Autodesk Inventor part; units mm, degrees
(part 2 of 2)
  line L793 (-106453, -86326.2124) -> (-106453, -83926.2124)
  line L794 (-106453, -83926.2124) -> (-106353, -83926.2124)
  line L795 (-106353, -83926.2124) -> (-106353, -90167.9126)
  line L796 (-106353, -90167.9126) -> (-97738.8492, -90167.9126)
  line L797 (-106453, -82706.2124) -> (-106353, -82706.2124)
  line L798 (-106353, -82706.2124) -> (-106353, -82456.2124)
  line L799 (-106453, -82706.2124) -> (-106453, -82206.2124)
  line L800 (-106353, -82456.2124) -> (-104713, -82456.2124)
  line L801 (-104713, -82456.2124) -> (-104713, -83516.2124)
  line L802 (-104713, -83516.2124) -> (-103563, -83516.2124)
  line L803 (-103563, -83516.2124) -> (-103563, -82456.2124)
  line L804 (-103563, -82456.2124) -> (-98350.4288, -82456.2124)
  line L805 (-97738.8492, -90167.9126) -> (-98350.4288, -82456.2124)
  line L806 (-106453, -82206.2124) -> (-104713, -82206.2124)
  line L807 (-104713, -82206.2124) -> (-104713, -82106.2124)
  line L808 (-104713, -82106.2124) -> (-103563, -82106.2124)
  line L809 (-103563, -82106.2124) -> (-103563, -82206.2124)
  line L810 (-103563, -82206.2124) -> (-101863, -82206.2124)
  line L811 (-107613, -65817.8595) -> (-107513, -65817.8595)
  line L812 (-107513, -65817.8595) -> (-107513, -65467.8595)
  line L813 (-107513, -65467.8595) -> (-104713, -65467.8595)
  line L814 (-104713, -65467.8595) -> (-104713, -66447.8595)
  line L815 (-104713, -66447.8595) -> (-103563, -66447.8595)
  line L816 (-103563, -66447.8595) -> (-103563, -65467.8595)
  line L817 (-107613, -67037.8595) -> (-107613, -67637.8595)
  line L818 (-107613, -67637.8595) -> (-108513, -70077.1217)
  line L819 (-107613, -67037.8595) -> (-107513, -67037.8595)
  line L820 (-107513, -67037.8595) -> (-107513, -70077.1217)
  line L821 (-108513, -70077.1217) -> (-108513, -71877.1217)
  line L822 (-101863, -82206.2124) -> (-101863, -81606.2124)
  line L823 (-101863, -81606.2124) -> (-101763, -81606.2124)
  line L824 (-101763, -81606.2124) -> (-101763, -82206.2124)
  line L825 (-101763, -82206.2124) -> (-98119.4702, -82206.2124)
  line L826 (-98365.317, -79106.2124) -> (-101763, -79106.2124)
  line L827 (-101763, -79106.2124) -> (-101763, -79706.2124)
  line L828 (-101763, -79706.2124) -> (-101863, -79706.2124)
  line L829 (-101963, -79106.2124) -> (-101963, -79056.2124)
  line L830 (-101963, -79056.2124) -> (-103013, -79056.2124)
  line L831 (-103013, -79056.2124) -> (-103013, -78956.2124)
  line L832 (-98635.9282, -78856.2124) -> (-99052.2817, -73606.2124)
  line L833 (-103963, -79056.2124) -> (-103963, -74806.2124)
  line L834 (-103963, -79056.2124) -> (-107463, -79056.2124)
  line L835 (-107463, -78956.2124) -> (-107463, -79056.2124)
  line L836 (-108413, -79056.2124) -> (-108513, -79056.2124)
  line L837 (-108513, -79056.2124) -> (-108513, -74016.2124)
  line L838 (-108413, -73606.2124) -> (-108413, -79056.2124)
  line L839 (-108513, -71877.1217) -> (-108413, -71877.1217)
  line L840 (-101863, -79106.2124) -> (-101963, -79106.2124)
  line L841 (-101863, -79706.2124) -> (-101863, -79106.2124)
  line L842 (-103013, -78956.2124) -> (-101963, -78956.2124)
  line L843 (-101963, -78956.2124) -> (-101963, -78856.2124)
  line L844 (-101963, -78856.2124) -> (-98635.9282, -78856.2124)
  line L845 (-107463, -78956.2124) -> (-104063, -78956.2124)
  line L846 (-108413, -73356.2124) -> (-108413, -73097.1217)
  line L847 (-108413, -73097.1217) -> (-108513, -73097.1217)
  line L848 (-108513, -73097.1217) -> (-108513, -74016.2124)
  line L849 (-108413, -73606.2124) -> (-104713, -73606.2124)
  line L850 (-104713, -73606.2124) -> (-104713, -74806.2124)
  line L851 (-104713, -74806.2124) -> (-103413, -74806.2124)
  line L852 (-104063, -74806.2124) -> (-104063, -78956.2124)
  line L853 (-103413, -74806.2124) -> (-103413, -73606.2124)
  line L854 (-103413, -73606.2124) -> (-99052.2817, -73606.2124)
  line L855 (-99072.108, -73356.2124) -> (-99697.6971, -65467.8595)
  line L856 (-104713, -70227.1217) -> (-104713, -73356.2124)
  line L857 (-107513, -70077.1217) -> (-104563, -70077.1217)
  line L858 (-108413, -71877.1217) -> (-108413, -70227.1217)
  line L859 (-108413, -70227.1217) -> (-104713, -70227.1217)
  line L860 (-108513, -70077.1217) -> (-107513, -70077.1217) construction
  line L861 (-104563, -70077.1217) -> (-104563, -73356.2124)
  line L862 (-99072.108, -73356.2124) -> (-104563, -73356.2124)
  line L863 (-104713, -73356.2124) -> (-108413, -73356.2124)
  line L864 (-99697.6971, -65467.8595) -> (-103563, -65467.8595)
  line L865 (-104613, -99029.6129) -> (-104613, -98659.6129)
  line L866 (-104613, -98659.6129) -> (-103653, -98659.6129)
  line L867 (-106353, -99029.6129) -> (-104613, -99029.6129)
  line L868 (-103653, -99029.6129) -> (-97036.0684, -99029.6129)
  line L869 (-103653, -98659.6129) -> (-103653, -99029.6129)
  line L870 (-92256.354, -106329.6129) -> (-92256.354, -78829.6129)
  line L871 (-96222.2151, -106129.6129) -> (-92456.354, -106129.6129)
  line L872 (-96206.354, -106329.6129) -> (-92256.354, -106329.6129)
  line L873 (-92456.354, -106129.6129) -> (-92456.354, -78877.5442)
  line L874 (-99463, -65217.8595) -> (-99178.2074, -65217.8595)
  line L875 (-99450.8774, -65417.8595) -> (-99300.8774, -65417.8595)
  line L876 (-92456.354, -78877.5442) -> (-99300.8774, -65417.8595)
  line L877 (-92256.354, -78829.6129) -> (-99178.2074, -65217.8595)
  line L878 (-92456.354, -99487.1129) -> (-93271.354, -99487.1129)
  line L879 (-93271.354, -99487.1129) -> (-93271.354, -98672.1129)
  line L880 (-93271.354, -98672.1129) -> (-92456.354, -98672.1129)
  line L881 (-92456.354, -98672.1129) -> (-92456.354, -99487.1129)
  line L882 (-92456.354, -99487.1129) -> (-93271.354, -98672.1129) construction
  line L883 (-93271.354, -99487.1129) -> (-92456.354, -98672.1129) construction
  line L884 (-92456.354, -90987.1129) -> (-93271.354, -90987.1129)
  line L885 (-93271.354, -90987.1129) -> (-93271.354, -90172.1129)
  line L886 (-93271.354, -90172.1129) -> (-92456.354, -90172.1129)
  line L887 (-92456.354, -90172.1129) -> (-92456.354, -90987.1129)
  line L888 (-92456.354, -82487.1129) -> (-93271.354, -82487.1129)
  line L889 (-93271.354, -82487.1129) -> (-93271.354, -81672.1129)
  line L890 (-93271.354, -81672.1129) -> (-92456.354, -81672.1129)
  line L891 (-92456.354, -81672.1129) -> (-92456.354, -82487.1129)
  line L892 (-48823, -52627.8595) -> (-48823, -52097.8595)
  line L893 (-48823, -52097.8595) -> (-42123, -52097.8595)
  line L894 (-42123, -52097.8595) -> (-42123, -52627.8595)
  line L895 (-38789.6466, -50375.6793) -> (-39177.876, -49986.0924)
  line L896 (-39177.876, -49986.0924) -> (-40629.9726, -51433.1291)
  line L897 (-40629.9726, -51433.1291) -> (-40241.7433, -51822.7161)
  line L898 (-42293, -30653.9912) -> (-42293, -30793.9912)
  line L899 (-116563, -42028.8644) -> (-116563, -42928.8644)
  line L900 (-49867.455, -28903.9912) -> (-50017.455, -28903.9912)
  line L901 (-36598.9321, -47509.4379) -> (-37304.8036, -46801.098)
  line L902 (-35746.9496, -45531.0228) -> (-35323.4267, -45956.0267)
  line L903 (-35323.4267, -45956.0267) -> (-36598.4384, -47226.5956)
  line L904 (-36598.4384, -47226.5956) -> (-37021.9613, -46801.5917)
  line L905 (-37021.9613, -46801.5917) -> (-35746.9496, -45531.0228)
  line L906 (-34282.1913, -40880.8096) -> (-37823.8905, -44410.1675)
  line L907 (-37823.8905, -44410.1675) -> (-37576.8354, -44658.0864)
  line L908 (-37576.8354, -44658.0864) -> (-34035.1362, -41128.7286)
  line L909 (-34035.1362, -41128.7286) -> (-34282.1913, -40880.8096)
  line L910 (-56758, -33963.9912) -> (-56758, -37333.9912)
  line L911 (-103963, -51867.8595) -> (-103963, -54717.8595)
  line L912 (-121383, -41348.8644) -> (-121533, -41348.8644)
  line L913 (-121383, -43318.8644) -> (-121533, -43318.8644)
  point P0 (-48088.5906, -37513.9912)
  point P1 (-116561.9399, -50418.8644)
  point P2 (-92863.854, -99079.6129)
  dimension "d18" = 12850
  dimension "d23" = 168175.668
  dimension "d30" = 19239.0056
  dimension "d35" = 25977.9567
  dimension "d420" = 2440
  dimension "d421" = 3610
  dimension "d422" = 134.9
  dimension "d425" = 23543
  dimension "d427" = 30793.9912
  dimension "d431" = 1120
  dimension "d432" = 750
  dimension "d436" = 2200
  dimension "d443" = 18750
  dimension "d444" = 13450
  dimension "d455" = 5400
  dimension "d466" = 1510
  dimension "d467" = 490
  dimension "d468" = 200
  dimension "d472" = 2050
  dimension "d474" = 180
  dimension "d478" = 650
  dimension "d485" = 2010
  dimension "d486" = 1600
  dimension "d488" = 2740
  dimension "d489" = 140
  dimension "d507" = 150
  dimension "d514" = 280
  dimension "d515" = 1370
  dimension "d516" = 1860
  dimension "d519" = 1040
  dimension "d555" = 140
  dimension "d566" = 1040
  dimension "d582" = 1000
  dimension "d598" = 140
  dimension "d605" = 140
  dimension "d606" = 140
  dimension "d611" = 1200
  dimension "d622" = 1750
  dimension "d623" = 1000
  dimension "d626" = 31200
  dimension "d627" = 150
  dimension "d628" = 150
  dimension "d635" = 280
  dimension "d669" = 4870
  dimension "d670" = 4300
  dimension "d690" = 794.4094
  dimension "d722" = 4750
  dimension "d725" = 1200
  dimension "d727" = 2450
  dimension "d730" = 100
  dimension "d734" = 1700
  dimension "d735" = 250
  dimension "d738" = 100
  dimension "d742" = 7338
  dimension "d754" = 1200
  dimension "d775" = 1800
  dimension "d776" = 1415
  dimension "d777" = 100
  dimension "d782" = 2860
  dimension "d783" = 150
  dimension "d784" = 150.9956
  dimension "d785" = 310
  dimension "d786" = 910
  dimension "d789" = 150
  constraints: 1821 end point, 415 perpendicular, 292 collinear, 210 horizontal, 197 vertical, 94 point on line, 59 equal length, 37 parallel, 9 point on circle, 6 midpoint, 4 centre point, 3 tangent, 2 coincident, 1 equal radius, 18 other
  measures "d18" distance of L4.start L4.end
  measures "d23" distance of L1.end L2.end
  measures "d30" distance between parallel lines of L0 L4
  measures "d35" distance from line of L1 L4.start
  measures "d420" distance of L6.end L7.end
  measures "d421" distance of L7.end L8.end
  measures "d422" angle of L8 L7
  measures "d425" distance from line of L1 L5.start
  measures "d427" distance from line of L0 L5.start
  measures "d431" distance between parallel lines of L8 L17
  measures "d432" distance of L16.end L17.end
  measures "d436" distance of L8.end L9.end
  measures "d443" distance of L5.start L5.end
  measures "d444" distance of L5.end L6.end
  measures "d455" distance of L15.end L16.end
  measures "d466" distance between parallel lines of L9 L20
  measures "d467" distance of L14.end L15.end
  measures "d468" distance of L12.end L13.end
  measures "d472" distance between parallel lines of L25 L24
  measures "d474" distance of L25.end L27.end
  measures "d478" distance of L24.end L26.end
  measures "d485" distance of L27.end L29.end
  measures "d486" distance of L29.end L30.end
  measures "d488" distance between parallel lines of L29 L34
  measures "d489" distance of L33.start L33.end
  measures "d507" distance of L30.end L31.end
  measures "d514" distance of L24.start L24.end
  measures "d515" distance of L31.end L32.end
  measures "d516" distance of L32.end L36.end
  measures "d519" distance between parallel lines of L39 L34
  measures "d555" distance of L45.start L45.end
  measures "d566" distance from line of L41 L45.start
  measures "d582" distance between parallel lines of L9 L10
  measures "d598" distance between parallel lines of L51 L12
  measures "d605" distance between parallel lines of L21 L5
  measures "d606" distance between parallel lines of L54 L55
  measures "d611" distance of L51.end L52.end
  measures "d622" distance of L19.start L19.end
  measures "d623" distance of L49.end L48.end
  measures "d626" distance of L49.start L49.end
  measures "d627" distance between parallel lines of L23 L50
  measures "d628" distance between parallel lines of L49 L22
  measures "d635" distance between parallel lines of L44 L42
  measures "d669" distance between parallel lines of L63 L30
  measures "d670" distance of L39.start L39.end
  measures "d690" distance between parallel lines of L33 L61
  measures "d722" distance of L26.end L28.end
  measures "d725" distance between parallel lines of L70 L67
  measures "d727" distance between parallel lines of L57 L33
  measures "d730" distance of L70.end L71.end
  measures "d734" distance of L65.end L66.end
  measures "d735" distance between parallel lines of L28 L73
  measures "d738" distance of L66.end L67.end
  measures "d742" distance of L69.end L73.end
  measures "d754" distance between parallel lines of L78 L72
  measures "d775" distance of L70.start L75.end
  measures "d776" distance of L70.start L70.end
  measures "d777" distance of L75.end L76.end
  measures "d782" distance of L63.end L64.end
  measures "d783" distance of L89.end L90.end
  measures "d784" distance between parallel lines of L64 L92
  measures "d785" distance of L64.end L89.end
  measures "d786" distance between parallel lines of L90 L94
  measures "d789" distance between parallel lines of L63 L93
extrude "BaseFloor" add sketch "Architecture" along normal blind 100 contours L12 L13 L14 L15 L16 L17 L20 L18 L9 L8 L7 L6 L5 | L5 L898 L21 L51 L52 L55 L49 L50 L900 L23 L22 L54 L53 L20 L17 L16 L15 L14 L13 L12 | L6 L25 L27 L29 L30 L31 L32 L36 L37 L35 L33 L34 A0 L45 L46 L38 L199 L42 L41 L61 L39 L40 L43 L44 L198 L62 L60 L59 A1 L58 L57 L56 L63 L64 L89 L90 L91 L92 L93 L94 L95 L96 L97 L98 L99 L127 L114 L112 L113 L115 L116 L117 L118 L119 L120 L128 L129 L121 L122 L123 L124 L125 L130 L131 L132 L149 L150 L138 L137 L136 L134 L135 L133 L139 L140 L141 L148 L143 L142 L146 L158 L159 L160 L145 L144 L147 L208 L200 L201 L207 L209 L157 L219 L220 L218 L217 L216 L215 L311 L313 L214 L221 L222 L223 L224 L312 L310 L225 L226 L315 L314 L357 L358 L359 L322 L321 L320 L319 L318 L317 L306 L307 L308 L309 L316 L361 L323 L324 L345 L344 L343 L342 L341 L340 L338 L335 L337 L336 L339 L363 L364 L365 L388 L386 L385 L393 L394 L395 L387 L354 L356 L355 L366 L367 L368 L369 L370 L371 L372 L373 L381 L382 L383 L384 L398 L396 L397 L378 L377 L374 L375 L376 L379 L380 L400 L401 L402 L411 L412 L413 L414 L415 L416 L417 L418 L419 L420 L421 L422 L426 L423 L424 L425 L410 L405 L404 L403 L406 L407 L408 L409 L435 L436 L441 L446 L447 L448 L449 L912 L433 L432 L431 L391 L392 L399 L152 L362 L326 L325 L360 L297 L296 L151 L126 L900 L48 L19 L898 | L6 L24 L26 L28 L65 L66 L67 L68 L69 L73 L74 L164 L165 L166 L167 L168 L169 L170 L171 L172 L173 L174 L175 L176 L177 L190 L188 L187 L186 L189 L77 L76 L75 L70 L71 L72 L85 L86 L87 L88 L181 L182 L185 L184 L183 L161 L81 L80 L79 L78 L82 L83 L84 L193 L191 L194 L195 L196 L197 L227 L228 L234 L235 L236 L237 L241 L242 L256 L251 L250 L249 L248 L247 L246 L252 L253 L254 L255 L257 L258 L259 L260 L261 L277 L275 L274 L273 L272 L271 L270 L276 L278 L281 L291 L290 L292 L293 L294 L427 L428 L429 L461 L911 L465 L466 L467 L552 L553 L554 L551 L577 L555 L556 L557 L558 L559 L560 L578 L562 L563 L567 L566 L565 L564 L569 L570 L568 L571 L572 L573 L574 L575 L576 L811 L812 L813 L814 L815 L816 L864 L855 L862 L861 L857 L820 L819 L817 L818 L821 L839 L858 L859 L856 L863 L846 L847 L848 L837 L836 L838 L849 L850 L851 L852 L845 L835 L834 L833 L853 L854 L832 L844 L843 L842 L831 L830 L829 L840 L841 L828 L827 L826 L766 L825 L824 L823 L822 L810 L809 L808 L807 L806 L799 L797 L798 L800 L801 L802 L803 L804 L805 L796 L795 L794 L793 L792 L786 L785 L787 L788 L789 L790 L791 L868 L869 L866 L865 L867 L783 L782 L777 L776 L773 L784 L774 L775 L778 L779 L780 L781 L769 L768 L767 L765 L764 L763 L762 L759 L741 L742 L743 L734 L735 L736 L740 L755 L749 L748 L747 L746 L745 L744 L733 L732 L731 L730 L729 L724 L720 L718 L721 L722 L723 L725 L726 L727 L728 L757 L756 L738 L739 L737 L716 L703 L702 L704 L713 L714 L715 L705 L701 L700 L699 L698 L697 L694 L688 L687 L673 L690 L668 L663 L662 L661 L664 L665 L666 L667 L672 L671 L660 L659 L658 L657 L656 L655 L654 L653 L652 L651 L650 L649 L634 L630 L648 L647 L646 L645 L644 L643 L642 L641 L640 L633 L632 L631 L629 L628 L584 L583 L582 L581 L580 L579 L608 L609 L627 L626 L625 L616 L615 L614 L607 L606 L605 L604 L603 L602 L601 L600 L599 L588 L589 L590 L594 L595 L598 L597 L596 L593 L592 L591 L587 L586 L585 L550 L549 L548 L547 L546 L539 L540 L541 L545 L544 L543 L542 L538 L537 L536 L535 L534 L533 L532 L531 L530 L529 L528 L527 L526 L525 L524 L523 L522 L521 L520 L519 L518 L517 L516 L515 L514 L513 L512 L511 L510 L509 L503 L504 L505 L506 L507 A3 L495 L494 L493 L492 L491 L490 L489 L488 L487 L486 L485 L484 L483 L482 L481 A2 L480 L479 L478 L477 L496 L497 L476 L475 L474 L473 L472 L471 L470 L469 L468 L460 L459 L442 L443 L444 L445 L455 L456 L457 L458 L454 L453 L899 L447 L446 L441 L436 L435 L409 L408 L407 L406 L403 L404 L405 L410 L425 L424 L423 L426 L422 L421 L420 L419 L418 L417 L416 L415 L414 L413 L412 L411 L402 L401 L400 L380 L379 L376 L375 L374 L377 L378 L397 L396 L398 L384 L383 L382 L381 L373 L372 L371 L370 L369 L368 L367 L366 L355 L356 L354 L387 L395 L394 L393 L385 L386 L388 L365 L364 L363 L339 L336 L337 L335 L338 L340 L341 L342 L343 L344 L345 L324 L323 L361 L316 L309 L308 L307 L306 L317 L318 L319 L320 L321 L322 L359 L358 L357 L314 L315 L226 L225 L310 L312 L224 L223 L222 L221 L214 L313 L311 L215 L216 L217 L218 L220 L219 L157 L209 L207 L201 L200 L208 L147 L144 L145 L160 L159 L158 L146 L142 L143 L148 L155 L154 L153 L156 L139 L133 L135 L134 L136 L137 L138 L150 L149 L132 L131 L130 L125 L124 L123 L122 L121 L129 L128 L120 L119 L118 L117 L116 L115 L113 L112 L114 L127 L99 L98 L97 L96 L95 L94 L93 L92 L91 L90 L89 L64 L63 L56 L57 L58 A1 L59 L60 L62 L198 L44 L43 L40 L39 L61 L41 L42 L199 L38 L46 L45 A0 L34 L33 L35 L37 L36 L32 L31 L30 L29 L27 L25 | L19 L48 L50 L49 L55 L52 L51 L21 | L6 L7 L8 L901 L11 L162 L178 L179 L180 L895 L896 L897 L163 L894 L893 L892 L279 L280 L295 L766 L826 L827 L828 L841 L840 L829 L830 L831 L842 L843 L844 L832 L854 L853 L851 L850 L849 L838 L836 L837 L848 L847 L846 L863 L856 L859 L858 L839 L821 L818 L817 L819 L820 L857 L861 L862 L855 L864 L816 L815 L814 L813 L812 L811 L576 L575 L574 L573 L572 L571 L568 L564 L565 L566 L567 L563 L562 L578 L560 L559 L558 L557 L561 L577 L551 L466 L430 L429 L428 L427 L294 L293 L292 L290 L291 L281 L278 L276 L270 L271 L272 L273 L274 L275 L277 L261 L260 L259 L258 L257 L255 L254 L253 L252 L246 L247 L248 L249 L250 L251 L256 L242 L241 L237 L236 L235 L234 L228 L227 L197 L196 L195 L194 L674 L238 L240 L239 L675 L193 L84 L83 L82 L78 L79 L80 L81 L161 L183 L184 L185 L182 L181 L88 L87 L86 L85 L72 L71 L70 L75 L76 L77 L189 L186 L187 L188 L190 L177 L176 L175 L174 L173 L172 L171 L170 L169 L168 L167 L166 L165 L164 L74 L73 L69 L68 L67 L66 L65 L28 L26 L24 | L9 L18 L10 L901 | L296 L297 L360 L152 | L162 L180 L179 L178 | L325 L326 L362 L152 | L162 L897 L896 L895 | L399 L392 L391 L431 L390 L389 | L163 L892 L893 L894 | L912 L450 L913 L434 | L874 L877 L870 L872 L766 L871 L873 L876 L875 L295 | L913 L451 L452 L453 L454 L458 L457 L456 L455 L445 L444 L443 L442 L459 L460 L468 L469 L470 L471 L472 L473 L474 L475 L476 L497 L496 L477 L478 L479 L480 A2 L481 L482 L483 L484 L485 L486 L487 L488 L489 L490 L491 L492 L493 L494 L495 A3 L507 L506 L505 L504 L503 L509 L510 L511 L512 L513 L514 L515 L516 L517 L518 L519 L520 L521 L522 L523 L524 L525 L526 L527 L528 L529 L530 L531 L532 L533 L534 L535 L536 L537 L538 L542 L543 L544 L545 L541 L540 L539 L546 L547 L548 L549 L550 L585 L586 L587 L591 L592 L593 L596 L597 L598 L595 L594 L590 L589 L588 L599 L600 L601 L602 L603 L604 L605 L606 L607 L614 L615 L616 L625 L626 L627 L609 L608 L579 L580 L581 L582 L583 L584 L628 L629 L631 L632 L633 L640 L641 L642 L643 L644 L645 L646 L647 L648 L630 L634 L649 L650 L651 L652 L653 L654 L655 L656 L657 L658 L659 L660 L671 L672 L667 L666 L665 L664 L661 L662 L663 L668 L690 L692 L691 L669 L670 L681 L682 L683 L684 L685 L706 L707 L696 L695 L689 L693 L687 L688 L694 L697 L698 L699 L700 L701 L705 L708 L709 L710 L704 L702 L703 L716 L737 L739 L738 L756 L757 L728 L727 L726 L725 L723 L722 L721 L718 L720 L724 L729 L730 L731 L732 L733 L744 L745 L746 L747 L748 L749 L755 L740 L736 L735 L734 L743 L742 L741 L759 L762 L763 L764 L765 L767 L768 L769 L781 L780 L779 L778 L775 L774 L784 L773 L776 L777 L782 L783 L867 L865 L866 L869 L868 L791 L790 L789 L788 L787 L785 L786 L792 L793 L794 L795 L796 L805 L804 L803 L802 L801 L800 L798 L797 L799 L806 L807 L808 L809 L810 L822 L823 L824 L825 L766 L761 L772 L771 L770 L760 L751 L750 L712 L754 L753 L752 L711 L758 L719 L717 L680 L679 L636 L676 L677 L678 L639 L638 L637 L635 L502 L501 L500 L499 | L449 L448 L899 L453 L452 L451 L450 | L875 L876 L873 L890 L889 L888 L886 L885 L884 L880 L879 L878 L871 L766 | L873 L888 L889 L890 | L761 L770 L771 L772 | L637 L638 L639 L636 | L878 L879 L880 L873 | L873 L884 L885 L886 | L678 L677 L676 L636 | L712 L752 L753 L754 | L717 L719 L758 L711 | L833 L834 L835 L845 L852 L851 | L675 L192 L674 L191 | L570 L569 L564 L568 | L156 L153 L910 L139 | L556 L555 L577 L561 | L554 L553 L552 L467 L466 L551 | L911 L462 L463 L464 | L693 L686 L692 L673 | L100 L101 L102 L103 | L104 L105 L106 L107 | L111 L110 L109 L108 | L202 L203 L204 L211 L212 L213 L206 L205 | L231 L232 L243 L244 L245 L233 L230 L229 | L264 L265 L267 L268 L269 L266 L263 L262 | L282 L289 L283 L284 L287 L285 L286 L288 | L298 L299 L300 L303 L304 L305 L302 L301 | L329 L330 L331 L332 L333 L334 L328 L327 | L348 L349 L350 L351 L352 L353 L347 L346 | L440 L439 L438 L437 | L613 L612 L611 L610 | L617 L618 L619 L620 | L621 L622 L623 L624 | L902 L903 L904 L905 | L909 L908 L907 L906
extrude "MainFloor" add sketch "Architecture" along normal blind 250 contours L6 L24 L26 L28 L65 L66 L67 L68 L69 L73 L74 L164 L165 L166 L167 L168 L169 L170 L171 L172 L173 L174 L175 L176 L177 L190 L188 L187 L186 L189 L77 L76 L75 L70 L71 L72 L85 L86 L87 L88 L181 L182 L185 L184 L183 L161 L81 L80 L79 L78 L82 L83 L84 L193 L191 L194 L195 L196 L197 L227 L228 L234 L235 L236 L237 L241 L242 L256 L251 L250 L249 L248 L247 L246 L252 L253 L254 L255 L257 L258 L259 L260 L261 L277 L275 L274 L273 L272 L271 L270 L276 L278 L281 L291 L290 L292 L293 L294 L427 L428 L429 L461 L911 L465 L466 L467 L552 L553 L554 L551 L577 L555 L556 L557 L558 L559 L560 L578 L562 L563 L567 L566 L565 L564 L569 L570 L568 L571 L572 L573 L574 L575 L576 L811 L812 L813 L814 L815 L816 L864 L855 L862 L861 L857 L820 L819 L817 L818 L821 L839 L858 L859 L856 L863 L846 L847 L848 L837 L836 L838 L849 L850 L851 L852 L845 L835 L834 L833 L853 L854 L832 L844 L843 L842 L831 L830 L829 L840 L841 L828 L827 L826 L766 L825 L824 L823 L822 L810 L809 L808 L807 L806 L799 L797 L798 L800 L801 L802 L803 L804 L805 L796 L795 L794 L793 L792 L786 L785 L787 L788 L789 L790 L791 L868 L869 L866 L865 L867 L783 L782 L777 L776 L773 L784 L774 L775 L778 L779 L780 L781 L769 L768 L767 L765 L764 L763 L762 L759 L741 L742 L743 L734 L735 L736 L740 L755 L749 L748 L747 L746 L745 L744 L733 L732 L731 L730 L729 L724 L720 L718 L721 L722 L723 L725 L726 L727 L728 L757 L756 L738 L739 L737 L716 L703 L702 L704 L713 L714 L715 L705 L701 L700 L699 L698 L697 L694 L688 L687 L673 L690 L668 L663 L662 L661 L664 L665 L666 L667 L672 L671 L660 L659 L658 L657 L656 L655 L654 L653 L652 L651 L650 L649 L634 L630 L648 L647 L646 L645 L644 L643 L642 L641 L640 L633 L632 L631 L629 L628 L584 L583 L582 L581 L580 L579 L608 L609 L627 L626 L625 L616 L615 L614 L607 L606 L605 L604 L603 L602 L601 L600 L599 L588 L589 L590 L594 L595 L598 L597 L596 L593 L592 L591 L587 L586 L585 L550 L549 L548 L547 L546 L539 L540 L541 L545 L544 L543 L542 L538 L537 L536 L535 L534 L533 L532 L531 L530 L529 L528 L527 L526 L525 L524 L523 L522 L521 L520 L519 L518 L517 L516 L515 L514 L513 L512 L511 L510 L509 L503 L504 L505 L506 L507 A3 L495 L494 L493 L492 L491 L490 L489 L488 L487 L486 L485 L484 L483 L482 L481 A2 L480 L479 L478 L477 L496 L497 L476 L475 L474 L473 L472 L471 L470 L469 L468 L460 L459 L442 L443 L444 L445 L455 L456 L457 L458 L454 L453 L899 L447 L446 L441 L436 L435 L409 L408 L407 L406 L403 L404 L405 L410 L425 L424 L423 L426 L422 L421 L420 L419 L418 L417 L416 L415 L414 L413 L412 L411 L402 L401 L400 L380 L379 L376 L375 L374 L377 L378 L397 L396 L398 L384 L383 L382 L381 L373 L372 L371 L370 L369 L368 L367 L366 L355 L356 L354 L387 L395 L394 L393 L385 L386 L388 L365 L364 L363 L339 L336 L337 L335 L338 L340 L341 L342 L343 L344 L345 L324 L323 L361 L316 L309 L308 L307 L306 L317 L318 L319 L320 L321 L322 L359 L358 L357 L314 L315 L226 L225 L310 L312 L224 L223 L222 L221 L214 L313 L311 L215 L216 L217 L218 L220 L219 L157 L209 L207 L201 L200 L208 L147 L144 L145 L160 L159 L158 L146 L142 L143 L148 L155 L154 L153 L156 L139 L133 L135 L134 L136 L137 L138 L150 L149 L132 L131 L130 L125 L124 L123 L122 L121 L129 L128 L120 L119 L118 L117 L116 L115 L113 L112 L114 L127 L99 L98 L97 L96 L95 L94 L93 L92 L91 L90 L89 L64 L63 L56 L57 L58 A1 L59 L60 L62 L198 L44 L43 L40 L39 L61 L41 L42 L199 L38 L46 L45 A0 L34 L33 L35 L37 L36 L32 L31 L30 L29 L27 L25 | L570 L569 L564 L568 | L556 L555 L577 L561
extrude "GrassContainer" add sketch "Architecture" along normal blind 1150 contours L5 L898 L21 L51 L52 L55 L49 L50 L900 L23 L22 L54 L53 L20 L17 L16 L15 L14 L13 L12 | L9 L18 L10 L901
extrude "Grass" add sketch "Architecture" along normal blind 1000 contours L19 L48 L50 L49 L55 L52 L51 L21 | L902 L903 L904 L905 | L909 L908 L907 L906
extrude "Railings" add sketch "Architecture" along normal blind 1250 contours L912 L450 L913 L434 | L874 L877 L870 L872 L766 L871 L873 L876 L875 L295 | L675 L192 L674 L191 | L156 L153 L910 L139 | L911 L462 L463 L464 | L693 L686 L692 L673
extrude "Walls" add sketch "Architecture" along normal blind 3250 contours L6 L25 L27 L29 L30 L31 L32 L36 L37 L35 L33 L34 A0 L45 L46 L38 L199 L42 L41 L61 L39 L40 L43 L44 L198 L62 L60 L59 A1 L58 L57 L56 L63 L64 L89 L90 L91 L92 L93 L94 L95 L96 L97 L98 L99 L127 L114 L112 L113 L115 L116 L117 L118 L119 L120 L128 L129 L121 L122 L123 L124 L125 L130 L131 L132 L149 L150 L138 L137 L136 L134 L135 L133 L139 L140 L141 L148 L143 L142 L146 L158 L159 L160 L145 L144 L147 L208 L200 L201 L207 L209 L157 L219 L220 L218 L217 L216 L215 L311 L313 L214 L221 L222 L223 L224 L312 L310 L225 L226 L315 L314 L357 L358 L359 L322 L321 L320 L319 L318 L317 L306 L307 L308 L309 L316 L361 L323 L324 L345 L344 L343 L342 L341 L340 L338 L335 L337 L336 L339 L363 L364 L365 L388 L386 L385 L393 L394 L395 L387 L354 L356 L355 L366 L367 L368 L369 L370 L371 L372 L373 L381 L382 L383 L384 L398 L396 L397 L378 L377 L374 L375 L376 L379 L380 L400 L401 L402 L411 L412 L413 L414 L415 L416 L417 L418 L419 L420 L421 L422 L426 L423 L424 L425 L410 L405 L404 L403 L406 L407 L408 L409 L435 L436 L441 L446 L447 L448 L449 L912 L433 L432 L431 L391 L392 L399 L152 L362 L326 L325 L360 L297 L296 L151 L126 L900 L48 L19 L898 | L6 L7 L8 L901 L11 L162 L178 L179 L180 L895 L896 L897 L163 L894 L893 L892 L279 L280 L295 L766 L826 L827 L828 L841 L840 L829 L830 L831 L842 L843 L844 L832 L854 L853 L851 L850 L849 L838 L836 L837 L848 L847 L846 L863 L856 L859 L858 L839 L821 L818 L817 L819 L820 L857 L861 L862 L855 L864 L816 L815 L814 L813 L812 L811 L576 L575 L574 L573 L572 L571 L568 L564 L565 L566 L567 L563 L562 L578 L560 L559 L558 L557 L561 L577 L551 L466 L430 L429 L428 L427 L294 L293 L292 L290 L291 L281 L278 L276 L270 L271 L272 L273 L274 L275 L277 L261 L260 L259 L258 L257 L255 L254 L253 L252 L246 L247 L248 L249 L250 L251 L256 L242 L241 L237 L236 L235 L234 L228 L227 L197 L196 L195 L194 L674 L238 L240 L239 L675 L193 L84 L83 L82 L78 L79 L80 L81 L161 L183 L184 L185 L182 L181 L88 L87 L86 L85 L72 L71 L70 L75 L76 L77 L189 L186 L187 L188 L190 L177 L176 L175 L174 L173 L172 L171 L170 L169 L168 L167 L166 L165 L164 L74 L73 L69 L68 L67 L66 L65 L28 L26 L24 | L913 L451 L452 L453 L454 L458 L457 L456 L455 L445 L444 L443 L442 L459 L460 L468 L469 L470 L471 L472 L473 L474 L475 L476 L497 L496 L477 L478 L479 L480 A2 L481 L482 L483 L484 L485 L486 L487 L488 L489 L490 L491 L492 L493 L494 L495 A3 L507 L506 L505 L504 L503 L509 L510 L511 L512 L513 L514 L515 L516 L517 L518 L519 L520 L521 L522 L523 L524 L525 L526 L527 L528 L529 L530 L531 L532 L533 L534 L535 L536 L537 L538 L542 L543 L544 L545 L541 L540 L539 L546 L547 L548 L549 L550 L585 L586 L587 L591 L592 L593 L596 L597 L598 L595 L594 L590 L589 L588 L599 L600 L601 L602 L603 L604 L605 L606 L607 L614 L615 L616 L625 L626 L627 L609 L608 L579 L580 L581 L582 L583 L584 L628 L629 L631 L632 L633 L640 L641 L642 L643 L644 L645 L646 L647 L648 L630 L634 L649 L650 L651 L652 L653 L654 L655 L656 L657 L658 L659 L660 L671 L672 L667 L666 L665 L664 L661 L662 L663 L668 L690 L692 L691 L669 L670 L681 L682 L683 L684 L685 L706 L707 L696 L695 L689 L693 L687 L688 L694 L697 L698 L699 L700 L701 L705 L708 L709 L710 L704 L702 L703 L716 L737 L739 L738 L756 L757 L728 L727 L726 L725 L723 L722 L721 L718 L720 L724 L729 L730 L731 L732 L733 L744 L745 L746 L747 L748 L749 L755 L740 L736 L735 L734 L743 L742 L741 L759 L762 L763 L764 L765 L767 L768 L769 L781 L780 L779 L778 L775 L774 L784 L773 L776 L777 L782 L783 L867 L865 L866 L869 L868 L791 L790 L789 L788 L787 L785 L786 L792 L793 L794 L795 L796 L805 L804 L803 L802 L801 L800 L798 L797 L799 L806 L807 L808 L809 L810 L822 L823 L824 L825 L766 L761 L772 L771 L770 L760 L751 L750 L712 L754 L753 L752 L711 L758 L719 L717 L680 L679 L636 L676 L677 L678 L639 L638 L637 L635 L502 L501 L500 L499 | L873 L888 L889 L890 | L878 L879 L880 L873 | L873 L884 L885 L886 | L833 L834 L835 L845 L852 L851 | L100 L101 L102 L103 | L104 L105 L106 L107 | L111 L110 L109 L108 | L202 L203 L204 L211 L212 L213 L206 L205 | L231 L232 L243 L244 L245 L233 L230 L229 | L264 L265 L267 L268 L269 L266 L263 L262 | L282 L289 L283 L284 L287 L285 L286 L288 | L298 L299 L300 L303 L304 L305 L302 L301 | L329 L330 L331 L332 L333 L334 L328 L327 | L348 L349 L350 L351 L352 L353 L347 L346 | L440 L439 L438 L437 | L613 L612 L611 L610 | L617 L618 L619 L620 | L621 L622 L623 L624
extrude "UVG-MastersDesk" add sketch "Architecture" along normal blind 1350 contours L554 L553 L552 L467 L466 L551
sketch "Sketch2" plane through (0, 250, 0) normal (0, 1, 0) x (1, 0, 0)
  line L0 (54388, 31203.9912) -> (54438, 31203.9912)
  line L1 (54438, 31203.9912) -> (54438, 41193.9912)
  line L2 (54388, 31203.9912) -> (54388, 41193.9912)
  arc A0 (56438, 43243.9912) -> (54388, 41193.9912) centre (56438, 41193.9912) ccw
  line L3 (56438, 43243.9912) -> (61093, 43243.9912)
  arc A1 (62479.5243, 42852.3203) -> (61093, 43243.9912) centre (61093, 40593.9912) ccw
  line L4 (62479.5243, 42852.3203) -> (69082.6366, 38798.272)
  arc A2 (69082.6366, 38798.272) -> (70443, 38413.9912) centre (70443, 41013.9912) ccw
  line L5 (70443, 38413.9912) -> (104816.7449, 38413.9912)
  arc A3 (56438, 43193.9912) -> (54438, 41193.9912) centre (56438, 41193.9912) ccw
  line L6 (56438, 43193.9912) -> (61093, 43193.9912)
  arc A4 (62453.3634, 42809.7104) -> (61093, 43193.9912) centre (61093, 40593.9912) ccw
  line L7 (62453.3634, 42809.7104) -> (69056.4757, 38755.6621)
  arc A5 (69056.4757, 38755.6621) -> (70443, 38363.9912) centre (70443, 41013.9912) ccw
  line L8 (70443, 38363.9912) -> (104816.7449, 38363.9912)
  line L9 (110757.6536, 59968.8644) -> (121973, 59968.8644)
  line L10 (121973, 59968.8644) -> (121973, 59918.8644)
  line L11 (121973, 59918.8644) -> (110757.6536, 59918.8644)
  line L12 (52313, 31613.9912) -> (52313, 32133.9912) projected
  line L13 (52313, 31873.9912) -> (56513, 31873.9912) construction
  line L14 (56513, 33963.9912) -> (56513, 31613.9912) projected
  line L15 (54413, 31873.9912) -> (54413, 31203.9912) construction
  line L16 (56513, 29203.9912) -> (52313, 29203.9912) projected
  line L17 (53223, 44243.9912) -> (61093, 44243.9912) projected
  line L18 (60713, 42193.9912) -> (56513, 42193.9912) projected
  line L19 (58593, 42193.9912) -> (58593, 44243.9912) construction
  line L20 (59093, 43193.9912) -> (59093, 43243.9912) construction
  line L21 (58593, 43218.9912) -> (59093, 43218.9912)
  line L22 (61093, 44243.9912) -> (61093, 40593.9912)
  line L23 (81306.2965, 39883.9912) -> (82906.2965, 39883.9912) projected
  line L24 (82106.2965, 39883.9912) -> (82106.2965, 36893.9912) construction
  line L25 (83243, 36893.9912) -> (79883, 36893.9912) projected
  line L26 (82606.2965, 38413.9912) -> (82606.2965, 38363.9912) construction
  line L27 (82106.2965, 38388.9912) -> (82606.2965, 38388.9912) construction
  line L28 (70443, 43483.9912) -> (70443, 39883.9912) projected
  line L29 (104613, 39883.9912) -> (104613, 43633.9912) projected
  line L30 (109293, 41348.8644) -> (109293, 38948.8644) projected
  line L31 (103332.8895, 39883.9912) -> (104613, 39883.9912) projected
  line L32 (118183, 62318.8644) -> (119323, 62318.8644) projected
  line L33 (118753, 62318.8644) -> (118753, 57568.8644) construction
  line L34 (119253, 59968.8644) -> (119253, 59918.8644) construction
  line L35 (118753, 59943.8644) -> (119253, 59943.8644)
  line L36 (124773, 61418.8644) -> (124773, 57818.8644) projected
  line L37 (123873, 57568.8644) -> (117293, 57568.8644) projected
  line L38 (110993, 56618.8644) -> (110993, 57818.8644) projected
  line L39 (106343, 56717.8595) -> (103963, 56717.8595) projected
  line L40 (106343, 56717.8595) -> (110843, 56717.8595) construction
  line L41 (110843, 57818.8644) -> (110843, 53418.8644) projected
  line L42 (109293, 41348.8644) -> (104613, 41348.8644) construction
  line L43 (108768.944, 58131.0763) -> (106855.1723, 40196.474)
  line L44 (108719.2262, 58136.3816) -> (106805.4545, 40201.7793)
  arc A6 (104816.7449, 38363.9912) -> (106855.1723, 40196.474) centre (104816.7449, 40413.9912) ccw
  arc A7 (104816.7449, 38413.9912) -> (106805.4545, 40201.7793) centre (104816.7449, 40413.9912) ccw
  line L45 (108631.1221, 56839.5012) -> (108581.4044, 56844.8065) construction
  line L46 (108604.5956, 56590.9125) -> (108554.8779, 56596.2178) construction
  line L47 (108579.7368, 56593.5652) -> (108606.2632, 56842.1539) construction
  arc A8 (110757.6536, 59918.8644) -> (108768.944, 58131.0763) centre (110757.6536, 57918.8644) ccw
  arc A9 (110757.6536, 59968.8644) -> (108719.2262, 58136.3816) centre (110757.6536, 57918.8644) ccw
  line L48 (106964.5956, 41221.9174) -> (106914.8779, 41227.2227) construction
  line L49 (106991.1221, 41470.5061) -> (106941.4044, 41475.8114) construction
  line L50 (106966.2632, 41473.1588) -> (106939.7368, 41224.5701) construction
  point P0 (0, 0)
  point P1 (108593, 56717.8595)
  point P2 (106953, 41348.8644)
  dimension "d3195" = 50
  dimension "d3196" = 2000
  dimension "d3198" = 2600
  dimension "d3199" = 2500
  dimension "d3200" = 500
  dimension "d3201" = 500
  dimension "d3204" = 500
  dimension "d3205" = 2800
  dimension "d3214" = 250
  dimension "d3216" = 250
  dimension "d3217" = 2000
  dimension "d3218" = 2000
  dimension "d3219" = 2000
  constraints: 68 end point, 22 point on line, 20 point on circle, 20 tangent, 19 midpoint, 12 perpendicular, 10 centre point, 9 horizontal, 5 concentric, 5 vertical, 4 parallel, 1 equal radius
  measures "d3195" distance of L0.start L0.end
  measures "d3196" distance between parallel lines of L16 L0
  measures "d3198" radius of A4
  measures "d3199" distance between parallel lines of L22 L19
  measures "d3200" distance between parallel lines of L19 L20
  measures "d3201" distance between parallel lines of L24 L26
  measures "d3204" distance between parallel lines of L33 L34
  measures "d3205" distance between parallel lines of L36 L10
  measures "d3214" distance between parallel lines of L46 L45
  measures "d3216" distance between parallel lines of L48 L49
  measures "d3217" radius of A7
  measures "d3218" radius of A8
  measures "d3219" radius of A3
extrude "NavPath" add sketch "Sketch2" along normal blind 300 separate body
